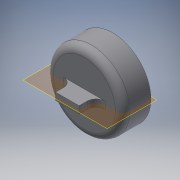
# Autodesk Inventor part: coupler
Saved by Autodesk Inventor 2017 (Build 210142000, 142)
## iProperties
Created: 2018-11-25
Part Number: coupler
Material: Generic
Document SubType Name: Modeling
Designer: Eric the Great
Density: 1 g/cm^3
Appearance: Default
Author: Eric the Great
Autodesk Inventor part; units mm, degrees
ref_plane "YZ Plane" through (0, 0, 0) normal (1, 0, 0) x (0, 1, 0)
ref_plane "XZ Plane" through (0, 0, 0) normal (0, 1, 0) x (-1, 0, 0)
ref_plane "XY Plane" through (0, 0, 0) normal (0, 0, 1) x (1, 0, 0)
sketch "Sketch1" plane through (0, 0, 0) normal (0, 0, 1) x (1, 0, 0)
  circle A0 centre (0, 0) radius 11 projected
  circle A1 centre (0, 0) radius 13.5
  point P0 (0, 0)
  dimension "d14" = 2.5
  constraints: 1 centre point, 1 coincident
  measures "d14" radial gap between concentric circles of A0 A1
ref_plane "Work Plane1" through (-19.2247, -19.2247, -7) normal (0, 0, -1) x (0, 1, 0)
extrude "Extrusion2" add sketch "Sketch1" against normal up to surface (7 mm away)
sketch "Sketch2" plane through (0, 0, 0) normal (0, 0, 1) x (1, 0, 0)
  circle A0 centre (0, 0) radius 11 projected
  circle A1 centre (0, 0) radius 13.5 projected
  point P0 (0, 0)
extrude "Extrusion3" add sketch "Sketch2" along normal blind 3 contours A0 | A1
sketch "Sketch3" plane through (0, 0, 3) normal (0, 0, 1) x (1, 0, 0)
  line L0 (-4.1456, -1.27) -> (4.1456, -1.27)
  line L1 (4.1456, -1.27) -> (4.1456, 1.27)
  line L2 (4.1456, 1.27) -> (-4.1456, 1.27)
  line L3 (-4.1456, 1.27) -> (-4.1456, -1.27)
  line L4 (-4.1456, -1.27) -> (4.1456, 1.27) construction
  line L5 (4.1456, -1.27) -> (-4.1456, 1.27) construction
  circle A0 centre (0, 0) radius 13.5 projected
  point P0 (0, 0)
  dimension "d10" = 2.54
  constraints: 12 end point, 3 midpoint, 2 parallel, 1 coincident, 1 horizontal, 1 perpendicular
  measures "d10" distance of L0.end L1.end
extrude "Extrusion4" add sketch "Sketch3" along normal blind 8 contours L3 L2 L1 L0
fillet "Fillet1" radius 3.175 2 edges at (-4.1456, 0, 3) (4.1456, 0, 3)
fillet "Fillet2" radius 2.54 1 edges at (-13.5, 0, 3)
ref_plane "Work Plane2" through (0, 0, 43.7679) normal (0, 1, 0) x (0, 0, 1)
body "Solid2"
